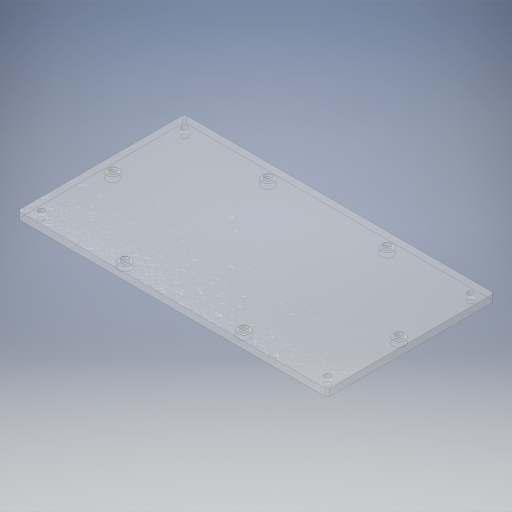
# Autodesk Inventor part: BT004_trajan20_21
Saved by Autodesk Inventor 2023 (Build 270158000, 158)
## iProperties
Company: HTBLA Kaindorf
RuleStatus: InUse
Created: 2022-08-07
Part Number: BT004_trajan20_21
Project: Zeichenmaschine_v2
Material: Acryl
Description: Hauptplatte unten
Document SubType Name: Modeling
Designer: trajan20
Density: 1.188 g/cm^3
Appearance: Transparent - farblos
Mass: 256.297 g
Surface Area: 784.687 cm^2
Volume: 215.738 cm^3
AfterDocNew0: iProperties-Editor_aufrufen
Author: jan
Keywords: 2021
Autodesk Inventor part; units mm, degrees
derived "BT000_trajan20_22_Zeichenmaschine_neu_Masterskizze.ipt"
sketch "Skizze4" plane through (0, 0, 0) normal (0, 0, 1) x (1, 0, 0)
  line L0 (0, 0) -> (-140, 0)
  line L1 (-140, 0) -> (-140, 260)
  line L2 (-140, 260) -> (0, 260)
  line L3 (0, 260) -> (0, 0)
  point P0 (-10, 80)
  point P1 (-70, 10)
  point P2 (-130, 80)
  point P3 (-70, 0)
  point P4 (-130, 10)
  point P5 (-10, 10)
  dimension "d6" = 140
  dimension "d7" = 260
  dimension "d33" = 80
  dimension "d34" = 10
  dimension "d35" = 10
  dimension "d36" = 10
  constraints: 8 end point, 3 horizontal alignment, 3 vertical alignment, 2 parallel, 1 horizontal, 1 midpoint, 1 perpendicular
  measures "d6" distance between parallel lines of L1 L3
  measures "d7" distance between parallel lines of L2 L0
  measures "d33" distance from line of L0 point (-10, 80)
  measures "d34" distance from line of L0 point (-70, 10)
  measures "d35" distance from line of L3 point (-10, 80)
  measures "d36" distance from line of L1 point (-130, 80)
extrude "Extrusion3" add sketch "Skizze4" along normal blind 6
ref_plane "Arbeitsebene1" through (0, 130, 0) normal (0, -1, 0) x (1, 0, 0)
ref_plane "Arbeitsebene2" through (-70, 260, 0) normal (-1, 0, 0) x (0, -1, 0)
fillet "Rundung2" radius 2 4 edges at (0, 0, 3) (-140, 0, 3) (-140, 260, 3) (0, 260, 3)
hole "Bohrung2" at (-10, 80, 0) at (-70, 10, 0) at (-130, 80, 0) direction (0, 0, 1) diameter 5.5 end through all counterbore diameter 10 counterbore depth 4
ref_plane "Arbeitsebene7" through (0, 130, 6) normal (0, 1, 0) x (-1, 0, 0)
hole "Bohrung3" at (-130, 10, 0) at (-10, 10, 0) direction (0, 0, 1) diameter 5 end through all
mirror "Spiegeln3" about plane through (0, 130, 6) normal (0, 1, 0) of "Bohrung2", "Bohrung3"
equation "\"d6\" = Basis_Haupt_Breite_Profillänge + 4 * AluProfil_Abstand"
equation "\"d7\" = Basis_Haupt_Länge_Profillänge + 4 * AluProfil_Abstand"
equation "\"d34\" = AluProfil_Abstand"
equation "\"d35\" = AluProfil_Abstand"
equation "\"d36\" = AluProfil_Abstand"
equation "\"Basis_Haupt_Breite_Profillänge\" = 100"
equation "\"AluProfil_Abstand\" = 10"
equation "\"Basis_Haupt_Länge_Profillänge\" = 220"
